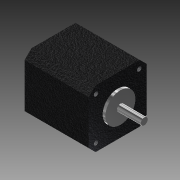
# Autodesk Inventor part: NEMA17-dual-shaft
Saved by Autodesk Inventor 2015 (Build 190159000, 159)
## iProperties
Created: 2013-07-10
Part Number: NEMA17-dual-shaft
Material: Generic
Document SubType Name: Modeling
Designer: Michael Green
Density: 1 g/cm^3
Appearance: Default
Author: Michael Green
Autodesk Inventor part; units mm, degrees
ref_plane "YZ Plane" through (0, 0, 0) normal (1, 0, 0) x (0, 1, 0)
ref_plane "XZ Plane" through (0, 0, 0) normal (0, 1, 0) x (-1, 0, 0)
ref_plane "XY Plane" through (0, 0, 0) normal (0, 0, 1) x (1, 0, 0)
sketch "Sketch1" plane through (0, 0, 0) normal (1, 0, 0) x (0, 1, 0)
  line L0 (0, 0) -> (42.3, 0)
  line L1 (42.3, 0) -> (42.3, 42.3)
  line L2 (42.3, 42.3) -> (0, 42.3)
  line L3 (0, 42.3) -> (0, 0)
  dimension "d0" = 42.3
  dimension "d1" = 42.3
  constraints: 8 end point, 2 parallel, 1 horizontal, 1 perpendicular
  measures "d0" distance of L2.end L1.end
  measures "d1" distance of L1.end L0.end
extrude "Extrusion1" add sketch "Sketch1" along normal blind 47
sketch "Sketch2" plane through (47, 0, 0) normal (1, 0, 0) x (0, 0, -1)
  circle A0 centre (-21.15, 21.15) radius 11
  dimension "d4" = 22
  constraints: 1 centre point, 1 coincident
  measures "d4" diameter of A0
extrude "Extrusion2" add sketch "Sketch2" along normal blind 2
sketch "Sketch3" plane through (47, 0, 0) normal (1, 0, 0) x (0, 0, -1)
  line L0 (-36.65, 5.3) -> (-5.65, 37) construction
  line L1 (-5.65, 5.3) -> (-36.65, 37) construction
  point P0 (-21.15, 21.15)
  point P1 (-21.15, 21.15)
  point P2 (-21.15, 21.15)
  dimension "d7" = 31
  constraints: 6 coincident, 4 end point, 2 midpoint
  measures "d7" distance of L1.end L0.end
hole "Hole1" at (47, 21.15, 21.15) at (47, 37, 36.65) at (47, 37, 5.65) at (47, 5.3, 5.65) at (47, 5.3, 36.65) direction (-1, 0, 0) diameter 3.242 depth 4.5 thread size "M4x0.7" class "6H" standard "ANSI Metric M Profile"
chamfer "Chamfer1" distance 5 angle 45 4 edges at (23.5, 42.3, 42.3) (23.5, 42.3, 0) (23.5, 0, 42.3) (23.5, 0, 0)
sketch "Sketch4" plane through (49, 21.15, 21.15) normal (1, 0, 0) x (0, 0, -1)
  circle A0 centre (0, 0) radius 11 projected
  circle A1 centre (0, 0) radius 2.5
  point P0 (21.15, -21.15)
  dimension "d18" = 5
  constraints: 1 centre point, 1 coincident
  measures "d18" diameter of A1
extrude "Extrusion3" add sketch "Sketch4" along normal blind 17.5 contours A1
sketch "Sketch5" plane through (0, 0, 0) normal (-1, 0, 0) x (0, 0, 1)
  circle A0 centre (21.15, 21.15) radius 2.5
  point P0 (0, 0)
  dimension "d21" = 5
  constraints: 1 centre point, 1 coincident
  measures "d21" diameter of A0
extrude "Extrusion4" add sketch "Sketch5" along normal blind 13
body "Solid1"
